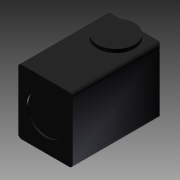
# Autodesk Inventor part: Shoulder
Saved by Autodesk Inventor 2012 (Build 160160000, 160)
## iProperties
Created: 2013-03-08
Part Number: Shoulder
Material: Default
Document SubType Name: Modeling
Designer: Andrew
Density: 1 g/cm^3
Author: Andrew
Autodesk Inventor part; units mm, degrees
ref_plane "YZ Plane" through (0, 0, 0) normal (1, 0, 0) x (0, 1, 0)
ref_plane "XZ Plane" through (0, 0, 0) normal (0, 1, 0) x (-1, 0, 0)
ref_plane "XY Plane" through (0, 0, 0) normal (0, 0, 1) x (1, 0, 0)
sketch "Sketch1" plane through (0, 0, 0) normal (0, 0, 1) x (1, 0, 0)
  line L0 (0, 0) -> (0, 41.5)
  circle A0 centre (0, 41.5) radius 11
  line L1 (0, 41.5) -> (0, 52.5)
  line L2 (0, 52.5) -> (16, 52.5)
  line L3 (16, 52.5) -> (16, 0)
  line L4 (16, 0) -> (0, 0)
  line L5 (0, 0) -> (-16, 0)
  line L6 (-16, 0) -> (-16, 52.5)
  line L7 (-16, 52.5) -> (0, 52.5)
  dimension "d1" = 22
  dimension "d0" = 41.5
  dimension "d2" = 16
  dimension "d3" = 16
  constraints: 16 end point, 4 perpendicular, 2 collinear, 1 coincident, 1 horizontal, 1 vertical, 1 vertical alignment, 2 other
  measures "d0" distance of L0.start L0.end
  measures "d2" distance of L1.end L2.end
  measures "d3" distance of L0.start L5.end
extrude "Extrusion1" add sketch "Sketch1" along normal mid plane 38
extrude "Extrusion2" add sketch "Sketch1" along normal mid plane 42 contours A0 L1 L0 | L0 L1 A0
fillet "Fillet1" radius 2 6 edges at (-16, 26.25, 19) (-16, 26.25, -19) (-16, 52.5, 0) (16, 52.5, 0) (16, 26.25, 19) (16, 26.25, -19)
sketch "Sketch2" plane through (-14, 0, 19) normal (0, -1, 0) x (1, 0, 0)
  circle A0 centre (14, -19) radius 11
  dimension "d9" = 22
  constraints: 1 centre point, 1 coincident
  measures "d9" diameter of A0
extrude "Extrusion3" cut sketch "Sketch2" against normal blind 1
body "Solid1"
